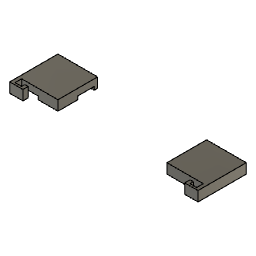
받침대 (Autodesk Fusion 360 design; units mm, degrees)
Autodesk Fusion 360 part; units mm, degrees
sketch "스케치1" plane through (0, 0, 0) normal (0, 0, 1) x (1, 0, 0)
  line L0 (-30, 30) -> (30, 30)
  line L1 (30, 30) -> (30, -30)
  line L2 (30, -30) -> (-30, -30)
  line L3 (-30, -30) -> (-30, 30)
  line L4 (-30, -30) -> (-10, -30)
  line L5 (-10, -30) -> (-10, -43)
  line L6 (-10, -43) -> (-30, -43)
  line L7 (-30, -43) -> (-30, -30)
  line L8 (-25, -30) -> (-25, -40)
  line L9 (-25, -40) -> (-10, -40)
  line L10 (-25, -30) -> (-25, 25)
  line L11 (-25, 25) -> (30, 25)
  line L12 (30, 0) -> (0, 0)
  line L13 (0, 0) -> (0, -30)
  line L14 (50, 60) -> (50, -50) construction
  line L15 (75, 30) -> (175, 30)
  line L16 (175, 30) -> (175, -30)
  line L17 (175, -30) -> (75, -30)
  line L18 (75, -30) -> (75, 30)
  line L19 (75, -30) -> (175, -30)
  line L20 (175, -30) -> (175, -75)
  line L21 (175, -75) -> (75, -75)
  line L22 (75, -75) -> (75, -30)
  line L23 (75, 25) -> (175, 25)
  line L24 (75, 0) -> (175, 0)
  dimension "d1" = 60
  dimension "d2" = 60
  dimension "d3" = 13
  dimension "d4" = 20
  dimension "d16" = 100
  dimension "d17" = 60
  dimension "d18" = 45
  constraint horizontal L0
  constraint vertical L1
  constraint horizontal L2
  constraint vertical L3
  constraint horizontal L4
  constraint vertical L5
  constraint horizontal L6
  constraint vertical L7
  constraint coincident L4 L8.start
  constraint perpendicular L4 L8
  constraint coincident L5 L9.end
  constraint perpendicular L5 L9
  constraint perpendicular L4 L10
  constraint coincident L1 L11.end
  constraint perpendicular L1 L11
  constraint midpoint L1 L12.start
  constraint coincident L12.end L13.start
  constraint perpendicular L1 L12
  constraint perpendicular L12 L13
  constraint perpendicular L0 L14
  constraint horizontal L15
  constraint vertical L16
  constraint horizontal L17
  constraint vertical L18
  constraint horizontal L19
  constraint vertical L20
  constraint horizontal L21
  constraint vertical L22
  constraint coincident L18 L23.start
  constraint perpendicular L18 L23
  constraint midpoint L18 L24.start
  constraint midpoint L16 L24.end
  measures "d1" distance of L0.start L2.end
  measures "d2" distance of L0.start L0.end
  measures "d3" distance of L2.end L6.end
  measures "d4" distance of L5.end L6.end
  measures "d16" distance of L15.start L15.end
  measures "d17" distance of L15.end L16.end
  measures "d18" distance of L19 L21
extrude "돌출1" add sketch "스케치1" along normal blind 10 contours L0 L1 L2 L3 L4 L10 L11 | L2 L4 L5 L6 L7 L8 L9 | L1 L2 L4 L10 L11 L12 L13 | L2 L4 L5 L8 L9 | L1 L2 L12 L13 makes body 1
extrude "돌출2" add sketch "스케치1" against normal blind 5 contours L0 L1 L2 L3 L4 L10 L11 | L2 L4 L5 L6 L7 L8 L9 | L1 L2 L12 L13 bodies 1
extrude "돌출3" cut sketch "스케치1" along normal blind 10 contours L2 L4 L5 L8 L9 bodies 1
sketch "스케치2" plane through (0, -43, 0) normal (0, -1, 0) x (1, 0, 0)
  line L0 (-10, -5) -> (-10, 10)
  line L1 (-10, 10) -> (-30, 10)
  line L2 (-30, 10) -> (-30, -5)
  line L3 (-30, -5) -> (-10, -5)
  line L4 (-15, 10) -> (-15, -5)
  constraint coincident L1 L4.start
  constraint coincident L3 L4.end
extrude "돌출4" add sketch "스케치2" along normal blind 5 from surface at -8 contours L0 L1 L3 L4 bodies 1
mirror "미러1" about plane through (0, 0, 0) normal (1, 0, 0) of bodies 1 makes body 2
move_body "이동1" bodies 2 to x (1, 0, 0) y (0, 1, 0) z (0, 0, 1) at (105, 0, 0)
move_body "이동2" bodies 2 to x (1, 0, 0) y (0, 1, 0) z (0, 0, 1) at (100, 0, 0)
move_body "이동3" bodies 2 to x (1, 0, 0) y (0, 1, 0) z (0, 0, 1) at (20, 0, 0)
extrude "돌출5" add sketch "스케치1" along normal blind 10 separate body contours L15 L16 L18 L23 | L16 L18 L23 L24 | L16 L17 L18 L19 L24 | L17 L19 L20 L21 L22 makes body 3
extrude "돌출6" add sketch "스케치1" against normal blind 5 contours L15 L16 L18 L23 | L16 L17 L18 L19 L24 bodies 3
extrude "돌출7" add sketch "스케치1" against normal blind 5 contours L17 L19 L20 L21 L22 bodies 3
hidden bodies 3
